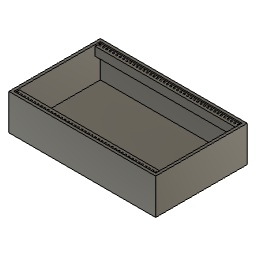
3U_Case (Autodesk Fusion 360 design; units mm, degrees)
Autodesk Fusion 360 part; units mm, degrees
sketch "Sketch2" plane through (0, 0, 0) normal (0, 0, 1) x (1, 0, 0)
  line L0 (110.68, 69) -> (-110.68, 69)
  line L1 (-110.68, 69) -> (-110.68, -69)
  line L2 (-110.68, -69) -> (110.68, -69)
  line L3 (110.68, -69) -> (110.68, 69)
  line L4 (110.68, 69) -> (-110.68, -69) construction
  line L5 (-110.68, 69) -> (110.68, -69) construction
  dimension "d14" = 138
  dimension "d15" = 221.36
  constraint horizontal L0
  constraint perpendicular L0 L1
  constraint parallel L0 L2
  constraint parallel L1 L3
  constraint coincident L4 origin
  constraint coincident L5 origin
  measures "d14" distance of L0.start L2.end
  measures "d15" distance of L0.start L0.end
extrude "Extrude2" add sketch "Sketch2" along normal blind 54
sketch "Sketch3" plane through (0, 0, 54) normal (0, 0, 1) x (-1, 0, 0)
  line L0 (-110.68, 69) -> (-110.68, -69)
  line L1 (-110.68, -69) -> (110.68, -69)
  line L2 (110.68, -69) -> (110.68, 69)
  line L3 (110.68, 69) -> (-110.68, 69)
  line L4 (-106.68, -65) -> (106.68, -65)
  line L5 (106.68, -65) -> (106.68, 65)
  line L6 (106.68, 65) -> (-106.68, 65)
  line L7 (-106.68, 65) -> (-106.68, -65)
  line L8 (-106.68, -65) -> (106.68, 65) construction
  line L9 (106.68, -65) -> (-106.68, 65) construction
  dimension "d18" = 130
  dimension "d19" = 213.36
  constraint horizontal L4
  constraint perpendicular L4 L5
  constraint parallel L4 L6
  constraint parallel L5 L7
  constraint coincident L8 origin
  constraint coincident L9 origin
  measures "d18" distance of L4.start L6.end
  measures "d19" distance of L4.start L4.end
extrude "Extrude3" cut sketch "Sketch3" against normal blind 50 contours L4 L5 L6 L7
sketch "Sketch4" plane through (0, 0, 54) normal (0, 0, 1) x (-1, 0, 0)
  line L0 (106.68, -65) -> (-106.68, -65)
  line L1 (-106.68, -65) -> (-106.68, 65)
  line L2 (-106.68, 65) -> (106.68, 65)
  line L3 (106.68, 65) -> (106.68, -65)
  line L4 (-110.68, 69) -> (-110.68, -69)
  line L5 (-110.68, -69) -> (110.68, -69)
  line L6 (110.68, -69) -> (110.68, 69)
  line L7 (110.68, 69) -> (-110.68, 69)
  line L8 (106.68, -65) -> (-106.68, -65)
  line L9 (-106.68, -65) -> (-106.68, -57)
  line L10 (-106.68, -57) -> (106.68, -57)
  line L11 (106.68, -57) -> (106.68, -65)
  dimension "d24" = 8
  dimension "d47" = 213.36
  constraint horizontal L8
  constraint vertical L9
  constraint horizontal L10
  constraint vertical L11
  constraint coincident L0.start L3.end
  measures "d24" distance of L0.start L10.end
  measures "d47" distance of L9.end L10.end
extrude "Extrude4" add sketch "Sketch4" along normal blind -20 and the other way blind 2 contours L0 L1 L3 L8 L9 L10 L11
chamfer "Chamfer1" distance 5 angle 45 1 edges at (0, 57, 34)
sketch "Sketch5" plane through (0, 0, 52) normal (0, 0, 1) x (-1, 0, 0)
  line L0 (106.68, -57) -> (-106.68, -57)
  line L1 (-106.68, -65) -> (106.68, -65)
  line L2 (106.68, -65) -> (106.68, -57)
  circle A0 centre (104.14, -62) radius 1.35
  line L3 (-106.68, -57) -> (-106.68, -65)
  dimension "d38" = 2.7
  dimension "d39" = 3
  dimension "d40" = 2.54
  measures "d38" diameter of A0
  measures "d39" distance of L1 A0.centre
  measures "d40" distance of L2 A0.centre
extrude "Extrude5" cut sketch "Sketch5" against normal blind 10 contours A0
pattern_linear "R-Pattern1" count 42 spacing 5.08 along (1, 0, 0) of "Extrude5"
mirror "Mirror2" about plane through (0, 0, 0) normal (0, 1, 0) of "Extrude4", "Chamfer1", "Extrude5", "R-Pattern1"
equation "_hp = 5.08 mm"
equation "case_width_hp = 42"
equation "side_wall_width = 4 mm"
equation "top_bottom_wall_width = 4 mm"
equation "case_depth = 50 mm"
equation "threeU_height = 130 mm"
equation "base_height = 4 mm"
equation "d14 = threeU_height + ( 2 * top_bottom_wall_width )"
equation "d15 = ( case_width_hp * _hp ) + ( 2 * side_wall_width )"
equation "d16 = case_depth + base_height"
equation "d18 = threeU_height"
equation "d19 = case_width_hp * _hp"
equation "d20 = -case_depth"
equation "rail_thickness = 8 mm"
equation "rail_depth = 20 mm"
equation "d25 = -rail_depth"
equation "d27 = rail_lip"
equation "rail_lip = 2 mm"
equation "screw_hole_diameter = 2.7 mm"
equation "screw_hole_spacing = 5.08 mm"
equation "screw_hole_depth = 10 mm"
equation "d40 = screw_hole_spacing / 2"
equation "d41 = -screw_hole_depth"
equation "d43 = case_width_hp"
equation "d45 = ( case_width_hp - 1 ) * _hp"
equation "d47 = case_width_hp * _hp"
equation "vent_slot_angle = 34 deg"
equation "vent_slot_ratio = 0.7"
equation "vent_slot_width = 3 mm"
